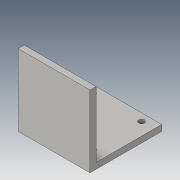
# Autodesk Inventor part: Y_carriage_90_bearing_mount
Saved by Autodesk Inventor 2016 (Build 200138000, 138)
## iProperties
Created: 2017-05-10
Part Number: Y_carriage_90_bearing_mount
Material: Generic
Document SubType Name: Modeling
Designer: Spark Electronics
Density: 1 g/cm^3
Appearance: Default
Author: Spark Electronics
Autodesk Inventor part; units mm, degrees
ref_plane "YZ Plane" through (0, 0, 0) normal (1, 0, 0) x (0, 1, 0)
ref_plane "XZ Plane" through (0, 0, 0) normal (0, 1, 0) x (-1, 0, 0)
ref_plane "XY Plane" through (0, 0, 0) normal (0, 0, 1) x (1, 0, 0)
sketch "Sketch1" plane through (0, 0, 0) normal (1, 0, 0) x (0, 1, 0)
  line L0 (-7.48, 28.2623) -> (30.52, 28.2623)
  line L1 (30.52, 28.2623) -> (30.52, 25.0623)
  line L2 (30.52, 25.0623) -> (-4.28, 25.0623)
  line L3 (-4.28, 25.0623) -> (-4.28, -9.7377)
  line L4 (-4.28, -9.7377) -> (-7.48, -9.7377)
  line L5 (-7.48, -9.7377) -> (-7.48, 28.2623)
  dimension "d0" = 3.2
  dimension "d1" = 38
  dimension "d2" = 3.2
  dimension "d3" = 38
  constraints: 12 end point, 5 perpendicular, 1 horizontal
  measures "d0" distance of L3.end L4.end
  measures "d1" distance between parallel lines of L0 L4
  measures "d2" distance of L0.end L1.end
  measures "d3" distance between parallel lines of L1 L5
extrude "Extrusion1" add sketch "Sketch1" along normal blind 38
sketch "Sketch2" plane through (0, -7.48, -9.7377) normal (0, -1, 0) x (1, 0, 0)
  circle A0 centre (5.3744, 30) radius 1.5
  line L0 (0, 0) -> (0, 38) projected
  line L1 (0, 0) -> (38, 0) projected
  line L2 (38, 38) -> (38, 0) projected
  line L3 (0, 38) -> (38, 38) projected
  circle A1 centre (5.3744, 4) radius 1.5
  circle A2 centre (31.3744, 30) radius 1.5
  circle A3 centre (31.3744, 4) radius 1.5
  dimension "d13" = 26
  dimension "d16" = 26
  dimension "d19" = 8
  dimension "d20" = 3
  constraints: 4 centre point, 1 horizontal, 1 vertical, 6 other
  measures "d13" distance of A0.centre A1.centre
  measures "d16" distance of A0.centre A2.centre
  measures "d19" distance from line of L3 A2.centre
  measures "d20" diameter of A0
extrude "Extrusion2" cut sketch "Sketch2" against normal up to next contours A0 | A1 | A2 | A3
body "Solid1"
